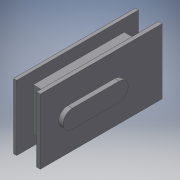
# Autodesk Inventor part: co2sensor
Saved by Autodesk Inventor 2019 (Build 230136000, 136)
## iProperties
Created: 2019-06-25
Part Number: co2sensor
Material: Generic
Document SubType Name: Modeling
Designer: Daniel
Density: 1 g/cm^3
Appearance: Default
Author: Daniel
Autodesk Inventor part; units mm, degrees
ref_plane "YZ Plane" through (0, 0, 0) normal (1, 0, 0) x (0, 1, 0)
ref_plane "XZ Plane" through (0, 0, 0) normal (0, 1, 0) x (-1, 0, 0)
ref_plane "XY Plane" through (0, 0, 0) normal (0, 0, 1) x (1, 0, 0)
sketch "Sketch1" plane through (0, 0, 0) normal (1, 0, 0) x (0, 1, 0)
  line L0 (0, 0) -> (36.957, 0)
  line L1 (36.957, 0) -> (36.957, -69.088)
  line L2 (36.957, -69.088) -> (0, -69.088)
  line L3 (0, -69.088) -> (0, 0)
  dimension "d0" = 69.088
  dimension "d1" = 36.957
  constraints: 8 end point, 2 parallel, 1 horizontal, 1 perpendicular
  measures "d0" distance of L2.end L0.start
  measures "d1" distance of L0.start L0.end
extrude "Extrusion1" add sketch "Sketch1" along normal blind 15.24
sketch "Sketch2" plane through (15.24, 0, 0) normal (1, 0, 0) x (0, 0, -1)
  line L0 (15.6183, 18.2767) -> (42.2027, 18.2767) construction
  line L1 (15.6183, 13.0907) -> (42.2027, 13.0907)
  line L2 (42.2027, 23.4628) -> (15.6183, 23.4628)
  arc A0 (15.6183, 23.4628) -> (15.6183, 13.0907) centre (15.6183, 18.2767) ccw
  arc A1 (42.2027, 13.0907) -> (42.2027, 23.4628) centre (42.2027, 18.2767) ccw
  point P0 (0, 0)
  point P1 (28.9105, 18.2767)
  constraints: 8 end point, 4 point on circle, 4 tangent, 2 centre point, 1 horizontal, 1 midpoint, 1 parallel
extrude "Extrusion2" add sketch "Sketch2" along normal blind 2.54
sketch "Sketch3" plane through (0, 0, -69.088) normal (0, 0, -1) x (-1, 0, 0)
  line L0 (-1.8203, -2.1906) -> (-13.1197, -2.1906)
  line L1 (-13.1197, -2.1906) -> (-13.1197, 2.4256)
  line L2 (-13.1197, 2.4256) -> (-1.8203, 2.4256)
  line L3 (-1.8203, 2.4256) -> (-1.8203, -2.1906)
  line L4 (-13.1197, 39.0109) -> (-1.8203, 39.0109)
  line L5 (-1.8203, 39.0109) -> (-1.8203, 33.2923)
  line L6 (-1.8203, 33.2923) -> (-13.1197, 33.2923)
  line L7 (-13.1197, 33.2923) -> (-13.1197, 39.0109)
  point P0 (0, 0)
  constraints: 16 end point, 4 parallel, 2 horizontal, 2 perpendicular, 2 point on line
extrude "Extrusion3" cut sketch "Sketch3" against normal blind 136.525
sketch "Sketch4" plane through (1.8203, 33.2923, -69.088) normal (0, 1, 0) x (1, 0, 0)
  line L0 (11.2994, 0) -> (11.2994, -69.088) projected
  line L1 (0, 0) -> (0, -69.088) projected
  line L2 (11.2994, 0) -> (0, 0)
  line L3 (0, 0) -> (0, -4.865)
  line L4 (0, -4.865) -> (11.2994, -4.865)
  line L5 (11.2994, -4.865) -> (11.2994, 0)
  line L6 (11.2994, -69.088) -> (13.4197, -69.088) projected
  line L7 (11.2994, -69.088) -> (0, -69.088)
  line L8 (0, -69.088) -> (0, -62.856)
  line L9 (0, -62.856) -> (11.2994, -62.856)
  line L10 (11.2994, -62.856) -> (11.2994, -69.088)
  point P0 (-1.8203, -69.088)
  constraints: 16 end point, 4 parallel, 2 horizontal, 2 perpendicular, 2 point on line
extrude "Extrusion4" cut sketch "Sketch4" against normal blind 136.525 contours L0 L4 L1 L2 | L0 L7 L1 L9
offset faces "Size1" outward -3.175 faces at (9.3532, 2.4256, -25.5623) (9.3532, 23.0034, -6.232) (5.5868, 33.2923, -44.8927) (5.5868, 23.0034, -64.223)
scale "Scale1" factors (0.7, 0.7, 0.7) then translate (0, 5.5436, -10.3632) bodies 1
body "Solid1"
